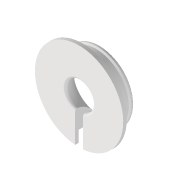
# Autodesk Inventor part: Buttomplate_BedholePlug
Saved by Autodesk Inventor 2021 (Build 250183000, 183)
## iProperties
Created: 2021-07-28
Part Number: Buttomplate_BedholePlug
Material: Generisch
Document SubType Name: Modeling
Designer: Rama
Density: 1 g/cm^3
Appearance: Vorgabe
Author: Rama
Autodesk Inventor part; units mm, degrees
ref_plane "YZ Plane" through (0, 0, 0) normal (1, 0, 0) x (0, 1, 0)
ref_plane "XZ Plane" through (0, 0, 0) normal (0, 1, 0) x (-1, 0, 0)
ref_plane "XY Plane" through (0, 0, 0) normal (0, 0, 1) x (1, 0, 0)
sketch "Skizze1" plane through (0, 0, 0) normal (0, 0, 1) x (1, 0, 0)
  circle A0 centre (0, 0) radius 7.45
  line L0 (-0.9, 9) -> (0.9, 9)
  line L1 (0.9, 9) -> (0.9, -9)
  line L2 (0.9, -9) -> (-0.9, -9)
  line L3 (-0.9, -9) -> (-0.9, 9)
  line L4 (-0.9, 9) -> (0.9, -9) construction
  line L5 (0.9, 9) -> (-0.9, -9) construction
  circle A1 centre (0, 0) radius 2.25
  point P0 (-0.9, -2.0622)
  point P1 (0.9, -2.0622)
  point P2 (0.9, -7.3954)
  point P3 (-0.9, -7.3954)
  dimension "d0" = 14.9
  dimension "d1" = 1.8
  dimension "d2" = 4.5
  constraints: 12 end point, 2 centre point, 2 coincident, 2 midpoint, 2 parallel, 1 horizontal, 1 perpendicular
  measures "d0" diameter of A0
  measures "d1" distance of L1.end L2.end
  measures "d2" diameter of A1
extrude "Extrusion1" add sketch "Skizze1" along normal blind 3 contours A0 L1 A1 | L1 A1 L3 A0 | L3 A1 A0 picked at (0.4002, 5.6965)
sketch "Skizze2" plane through (0, 0, 3) normal (0, 0, 1) x (1, 0, 0)
  line L0 (0.9, -2.0622) -> (0.9, -7.3954) projected
  arc A0 (0.9, -7.3954) -> (-0.9, -7.3954) centre (0, 0) ccw projected
  line L1 (-0.9, -7.3954) -> (-0.9, -2.0622) projected
  arc A1 (0.9, -2.0622) -> (-0.9, -2.0622) centre (0, 0) ccw projected
  circle A2 centre (0, 0) radius 10
  line L2 (-0.9, 11.3464) -> (0.9, 11.3464)
  line L3 (0.9, 11.3464) -> (0.9, -11.3464)
  line L4 (0.9, -11.3464) -> (-0.9, -11.3464)
  line L5 (-0.9, -11.3464) -> (-0.9, 11.3464)
  line L6 (-0.9, 11.3464) -> (0.9, -11.3464) construction
  line L7 (0.9, 11.3464) -> (-0.9, -11.3464) construction
  point P0 (-0.9, -9.9594)
  point P1 (-0.9, 2.0622)
  point P2 (-0.9, 7.3954)
  point P3 (0.9, 7.3954)
  point P4 (0.9, 2.0622)
  point P5 (0.9, -9.9594)
  dimension "d5" = 20
  dimension "d6" = 1.8
  constraints: 12 end point, 2 midpoint, 2 parallel, 1 centre point, 1 coincident, 1 horizontal, 1 perpendicular
  measures "d5" diameter of A2
  measures "d6" distance of L3.end L4.end
extrude "Extrusion2" add sketch "Skizze2" along normal blind 0.8 contours A1 L3 A0 L0 | A0 L3 A2 | A1 L5 A0 L3 | A0 L5 A2 L3 | A1 L1 A0 L5 | A0 L5 A2
sketch "Skizze3" plane through (0, 0, 0) normal (0, 0, -1) x (-1, 0, 0)
  line L0 (-0.9, -2.0622) -> (-0.9, -7.3954) projected
  arc A0 (0.9, -2.0622) -> (-0.9, -2.0622) centre (0, 0) ccw projected
  line L1 (0.9, -7.3954) -> (0.9, -2.0622) projected
  arc A1 (0.9, -7.3954) -> (-0.9, -7.3954) centre (0, 0) ccw projected
  circle A2 centre (0, 0) radius 7.75
  line L2 (0.9, 14.7103) -> (-0.9, 14.7103)
  line L3 (-0.9, 14.7103) -> (-0.9, -14.7103)
  line L4 (-0.9, -14.7103) -> (0.9, -14.7103)
  line L5 (0.9, -14.7103) -> (0.9, 14.7103)
  line L6 (0.9, 14.7103) -> (-0.9, -14.7103) construction
  line L7 (-0.9, 14.7103) -> (0.9, -14.7103) construction
  point P0 (-0.9, -7.6976)
  point P1 (0.9, -7.6976)
  dimension "d9" = 15.5
  dimension "d10" = 1.8
  constraints: 12 end point, 2 midpoint, 2 parallel, 1 centre point, 1 coincident, 1 horizontal, 1 perpendicular
  measures "d9" diameter of A2
  measures "d10" distance of L4.end L3.end
extrude "Extrusion3" add sketch "Skizze3" along normal blind 1.4 contours L0 A1 L3 A0 | L3 A2 A1 | L3 A1 L5 A0 | L3 A2 L5 A1 | L5 A1 L1 A0 | L5 A2 A1
sketch "Skizze4" plane through (0, 0, 3.8) normal (0, 0, 1) x (1, 0, 0)
  circle A0 centre (0, 0) radius 3
  constraints: 1 centre point, 1 coincident
extrude "Extrusion4" cut sketch "Skizze4" against normal through all
chamfer "Fase2" distance 0.3 angle 45 1 edges at (0, 7.75, 0)
fillet "Rundung5" radius 6 1 edges at (0, 3, -1.4)
chamfer "Fase3" distance 0.7 angle 45 1 edges at (0, 7.75, -1.4)
fillet "Rundung6" radius 0.5 1 edges at (0, 7.0754, -1.2194)
fillet "Rundung7" radius 0.2 1 edges at (0, 7.75, -0.7)
fillet "Rundung8" radius 0.5 1 edges at (0, 3, 3.8)
